Autodesk Inventor part; units mm, degrees
(part 2 of 4)
  line L887 (-15.9707, 10.3342) -> (-15.9954, 10.3717)
  line L888 (-15.9954, 10.3717) -> (-16.0287, 10.4125)
  line L889 (-16.0287, 10.4125) -> (-16.1438, 10.5298)
  line L890 (-16.1438, 10.5298) -> (-16.2774, 10.6739)
  line L891 (-16.2774, 10.6739) -> (-16.4262, 10.8486)
  line L892 (-16.4262, 10.8486) -> (-16.5875, 11.0549)
  line L893 (-16.5875, 11.0549) -> (-16.7591, 11.2943)
  line L894 (-16.7591, 11.2943) -> (-16.8478, 11.4265)
  line L895 (-16.8478, 11.4265) -> (-16.9387, 11.5685)
  line L896 (-16.9387, 11.5685) -> (-17.0299, 11.7175)
  line L897 (-17.0299, 11.7175) -> (-17.1238, 11.8785)
  line L898 (-17.1238, 11.8785) -> (-17.2101, 12.0338)
  arc A26 (-16.763, 12.6491) -> (-17.2101, 12.0338) centre (0, 0) ccw
  line L899 (-16.763, 12.6491) -> (-16.5887, 12.615)
  line L900 (-16.5887, 12.615) -> (-16.4066, 12.5755)
  line L901 (-16.4066, 12.5755) -> (-16.2367, 12.5348)
  line L902 (-16.2367, 12.5348) -> (-16.0735, 12.4922)
  line L903 (-16.0735, 12.4922) -> (-15.9204, 12.4487)
  line L904 (-15.9204, 12.4487) -> (-15.6397, 12.3595)
  line L905 (-15.6397, 12.3595) -> (-15.3936, 12.2698)
  line L906 (-15.3936, 12.2698) -> (-15.1815, 12.1823)
  line L907 (-15.1815, 12.1823) -> (-15.0031, 12.0998)
  line L908 (-15.0031, 12.0998) -> (-14.856, 12.0266)
  line L909 (-14.856, 12.0266) -> (-14.8069, 12.0075)
  line L910 (-14.8069, 12.0075) -> (-14.7636, 11.9956)
  line L911 (-14.7636, 11.9956) -> (-14.7265, 11.9906)
  line L912 (-14.7265, 11.9906) -> (-14.6957, 11.9923)
  line L913 (-14.6957, 11.9923) -> (-14.6716, 12.0004)
  line L914 (-14.6716, 12.0004) -> (-14.6544, 12.0147)
  line L915 (-14.6544, 12.0147) -> (-14.633, 12.0408)
  line L916 (-14.633, 12.0408) -> (-14.4097, 12.307)
  line L917 (-14.4097, 12.307) -> (-14.1816, 12.5693)
  line L918 (-14.1816, 12.5693) -> (-14.1592, 12.5944)
  line L919 (-14.1592, 12.5944) -> (-14.1478, 12.6137)
  line L920 (-14.1478, 12.6137) -> (-14.1436, 12.6387)
  line L921 (-14.1436, 12.6387) -> (-14.1467, 12.6694)
  line L922 (-14.1467, 12.6694) -> (-14.1574, 12.7053)
  line L923 (-14.1574, 12.7053) -> (-14.1759, 12.7462)
  line L924 (-14.1759, 12.7462) -> (-14.2025, 12.7918)
  line L925 (-14.2025, 12.7918) -> (-14.2978, 12.9256)
  line L926 (-14.2978, 12.9256) -> (-14.4072, 13.0888)
  line L927 (-14.4072, 13.0888) -> (-14.5269, 13.2846)
  line L928 (-14.5269, 13.2846) -> (-14.654, 13.5137)
  line L929 (-14.654, 13.5137) -> (-14.786, 13.777)
  line L930 (-14.786, 13.777) -> (-14.8529, 13.9214)
  line L931 (-14.8529, 13.9214) -> (-14.9205, 14.0759)
  line L932 (-14.9205, 14.0759) -> (-14.9872, 14.2373)
  line L933 (-14.9872, 14.2373) -> (-15.0547, 14.411)
  line L934 (-15.0547, 14.411) -> (-15.1157, 14.5779)
  arc A27 (-14.5779, 15.1157) -> (-15.1157, 14.5779) centre (0, 0) ccw
  line L935 (-14.5779, 15.1157) -> (-14.411, 15.0547)
  line L936 (-14.411, 15.0547) -> (-14.2373, 14.9872)
  line L937 (-14.2373, 14.9872) -> (-14.0759, 14.9205)
  line L938 (-14.0759, 14.9205) -> (-13.9214, 14.8528)
  line L939 (-13.9214, 14.8528) -> (-13.777, 14.786)
  line L940 (-13.777, 14.786) -> (-13.5137, 14.6539)
  line L941 (-13.5137, 14.6539) -> (-13.2846, 14.5269)
  line L942 (-13.2846, 14.5269) -> (-13.0888, 14.4072)
  line L943 (-13.0888, 14.4072) -> (-12.9256, 14.2978)
  line L944 (-12.9256, 14.2978) -> (-12.7918, 14.2025)
  line L945 (-12.7918, 14.2025) -> (-12.7462, 14.1759)
  line L946 (-12.7462, 14.1759) -> (-12.7053, 14.1574)
  line L947 (-12.7053, 14.1574) -> (-12.6694, 14.1467)
  line L948 (-12.6694, 14.1467) -> (-12.6387, 14.1436)
  line L949 (-12.6387, 14.1436) -> (-12.6137, 14.1478)
  line L950 (-12.6137, 14.1478) -> (-12.5944, 14.1592)
  line L951 (-12.5944, 14.1592) -> (-12.5693, 14.1816)
  line L952 (-12.5693, 14.1816) -> (-12.307, 14.4097)
  line L953 (-12.307, 14.4097) -> (-12.0408, 14.633)
  line L954 (-12.0408, 14.633) -> (-12.0147, 14.6544)
  line L955 (-12.0147, 14.6544) -> (-12.0004, 14.6716)
  line L956 (-12.0004, 14.6716) -> (-11.9923, 14.6957)
  line L957 (-11.9923, 14.6957) -> (-11.9906, 14.7264)
  line L958 (-11.9906, 14.7264) -> (-11.9956, 14.7636)
  line L959 (-11.9956, 14.7636) -> (-12.0075, 14.8069)
  line L960 (-12.0075, 14.8069) -> (-12.0266, 14.856)
  line L961 (-12.0266, 14.856) -> (-12.0998, 15.0031)
  line L962 (-12.0998, 15.0031) -> (-12.1823, 15.1815)
  line L963 (-12.1823, 15.1815) -> (-12.2698, 15.3936)
  line L964 (-12.2698, 15.3936) -> (-12.3595, 15.6397)
  line L965 (-12.3595, 15.6397) -> (-12.4487, 15.9204)
  line L966 (-12.4487, 15.9204) -> (-12.4922, 16.0735)
  line L967 (-12.4922, 16.0735) -> (-12.5348, 16.2367)
  line L968 (-12.5348, 16.2367) -> (-12.5755, 16.4066)
  line L969 (-12.5755, 16.4066) -> (-12.615, 16.5887)
  line L970 (-12.615, 16.5887) -> (-12.6491, 16.763)
  arc A28 (-12.0338, 17.2101) -> (-12.6491, 16.763) centre (0, 0) ccw
  line L971 (-12.0338, 17.2101) -> (-11.8785, 17.1238)
  line L972 (-11.8785, 17.1238) -> (-11.7175, 17.0299)
  line L973 (-11.7175, 17.0299) -> (-11.5685, 16.9387)
  line L974 (-11.5685, 16.9387) -> (-11.4265, 16.8478)
  line L975 (-11.4265, 16.8478) -> (-11.2943, 16.7591)
  line L976 (-11.2943, 16.7591) -> (-11.0549, 16.5875)
  line L977 (-11.0549, 16.5875) -> (-10.8486, 16.4262)
  line L978 (-10.8486, 16.4262) -> (-10.6739, 16.2774)
  line L979 (-10.6739, 16.2774) -> (-10.5298, 16.1438)
  line L980 (-10.5298, 16.1438) -> (-10.4125, 16.0287)
  line L981 (-10.4125, 16.0287) -> (-10.3717, 15.9954)
  line L982 (-10.3717, 15.9954) -> (-10.3342, 15.9707)
  line L983 (-10.3342, 15.9707) -> (-10.3004, 15.9544)
  line L984 (-10.3004, 15.9544) -> (-10.2706, 15.9466)
  line L985 (-10.2706, 15.9466) -> (-10.2452, 15.9468)
  line L986 (-10.2452, 15.9468) -> (-10.2244, 15.9551)
  line L987 (-10.2244, 15.9551) -> (-10.196, 15.9733)
  line L988 (-10.196, 15.9733) -> (-9.9013, 16.1575)
  line L989 (-9.9013, 16.1575) -> (-9.6034, 16.3364)
  line L990 (-9.6034, 16.3364) -> (-9.5743, 16.3534)
  line L991 (-9.5743, 16.3534) -> (-9.5575, 16.3682)
  line L992 (-9.5575, 16.3682) -> (-9.5457, 16.3908)
  line L993 (-9.5457, 16.3908) -> (-9.5392, 16.4209)
  line L994 (-9.5392, 16.4209) -> (-9.5383, 16.4584)
  line L995 (-9.5383, 16.4584) -> (-9.5433, 16.503)
  line L996 (-9.5433, 16.503) -> (-9.5545, 16.5545)
  line L997 (-9.5545, 16.5545) -> (-9.6038, 16.7112)
  line L998 (-9.6038, 16.7112) -> (-9.6574, 16.9003)
  line L999 (-9.6574, 16.9003) -> (-9.7107, 17.1235)
  line L1000 (-9.7107, 17.1235) -> (-9.7608, 17.3806)
  line L1001 (-9.7608, 17.3806) -> (-9.805, 17.6718)
  line L1002 (-9.805, 17.6718) -> (-9.8239, 17.8299)
  line L1003 (-9.8239, 17.8299) -> (-9.8405, 17.9976)
  line L1004 (-9.8405, 17.9976) -> (-9.8541, 18.1718)
  line L1005 (-9.8541, 18.1718) -> (-9.8647, 18.3579)
  line L1006 (-9.8647, 18.3579) -> (-9.8711, 18.5354)
  arc A29 (-9.1934, 18.8807) -> (-9.8711, 18.5354) centre (0, 0) ccw
  line L1007 (-9.1934, 18.8807) -> (-9.0535, 18.7712)
  line L1008 (-9.0535, 18.7712) -> (-8.9092, 18.6532)
  line L1009 (-8.9092, 18.6532) -> (-8.7763, 18.5399)
  line L1010 (-8.7763, 18.5399) -> (-8.6503, 18.4279)
  line L1011 (-8.6503, 18.4279) -> (-8.5336, 18.3196)
  line L1012 (-8.5336, 18.3196) -> (-8.3239, 18.1127)
  line L1013 (-8.3239, 18.1127) -> (-8.1454, 17.921)
  line L1014 (-8.1454, 17.921) -> (-7.9961, 17.7468)
  line L1015 (-7.9961, 17.7468) -> (-7.8747, 17.5923)
  line L1016 (-7.8747, 17.5923) -> (-7.7769, 17.4603)
  line L1017 (-7.7769, 17.4603) -> (-7.7418, 17.4209)
  line L1018 (-7.7418, 17.4209) -> (-7.7086, 17.3907)
  line L1019 (-7.7086, 17.3907) -> (-7.6778, 17.3693)
  line L1020 (-7.6778, 17.3693) -> (-7.6496, 17.3569)
  line L1021 (-7.6496, 17.3569) -> (-7.6244, 17.3532)
  line L1022 (-7.6244, 17.3532) -> (-7.6026, 17.3581)
  line L1023 (-7.6026, 17.3581) -> (-7.5717, 17.3716)
  line L1024 (-7.5717, 17.3716) -> (-7.2519, 17.5075)
  line L1025 (-7.2519, 17.5075) -> (-6.9296, 17.6376)
  line L1026 (-6.9296, 17.6376) -> (-6.8982, 17.6499)
  line L1027 (-6.8982, 17.6499) -> (-6.8793, 17.6618)
  line L1028 (-6.8793, 17.6618) -> (-6.8641, 17.6822)
  line L1029 (-6.8641, 17.6822) -> (-6.853, 17.711)
  line L1030 (-6.853, 17.711) -> (-6.8462, 17.7479)
  line L1031 (-6.8462, 17.7479) -> (-6.8442, 17.7927)
  line L1032 (-6.8442, 17.7927) -> (-6.8472, 17.8453)
  line L1033 (-6.8472, 17.8453) -> (-6.8714, 18.0078)
  line L1034 (-6.8714, 18.0078) -> (-6.8947, 18.203)
  line L1035 (-6.8947, 18.203) -> (-6.9124, 18.4318)
  line L1036 (-6.9124, 18.4318) -> (-6.9217, 18.6935)
  line L1037 (-6.9217, 18.6935) -> (-6.9198, 18.9881)
  line L1038 (-6.9198, 18.9881) -> (-6.9138, 19.1471)
  line L1039 (-6.9138, 19.1471) -> (-6.9039, 19.3155)
  line L1040 (-6.9039, 19.3155) -> (-6.8901, 19.4896)
  line L1041 (-6.8901, 19.4896) -> (-6.8714, 19.675)
  line L1042 (-6.8714, 19.675) -> (-6.85, 19.8514)
  arc A30 (-6.1266, 20.0864) -> (-6.85, 19.8514) centre (0, 0) ccw
  line L1043 (-6.1266, 20.0864) -> (-6.0056, 19.9563)
  line L1044 (-6.0056, 19.9563) -> (-5.8815, 19.8173)
  line L1045 (-5.8815, 19.8173) -> (-5.7679, 19.6846)
  line L1046 (-5.7679, 19.6846) -> (-5.661, 19.5542)
  line L1047 (-5.661, 19.5542) -> (-5.5627, 19.429)
  line L1048 (-5.5627, 19.429) -> (-5.388, 19.1918)
  line L1049 (-5.388, 19.1918) -> (-5.2416, 18.9746)
  line L1050 (-5.2416, 18.9746) -> (-5.1215, 18.7791)
  line L1051 (-5.1215, 18.7791) -> (-5.0257, 18.6076)
  line L1052 (-5.0257, 18.6076) -> (-4.9497, 18.4619)
  line L1053 (-4.9497, 18.4619) -> (-4.9212, 18.4175)
  line L1054 (-4.9212, 18.4175) -> (-4.8932, 18.3824)
  line L1055 (-4.8932, 18.3824) -> (-4.8661, 18.3566)
  line L1056 (-4.8661, 18.3566) -> (-4.8402, 18.3399)
  line L1057 (-4.8402, 18.3399) -> (-4.8159, 18.3323)
  line L1058 (-4.8159, 18.3323) -> (-4.7936, 18.3337)
  line L1059 (-4.7936, 18.3337) -> (-4.761, 18.3422)
  line L1060 (-4.761, 18.3422) -> (-4.4238, 18.4264)
  line L1061 (-4.4238, 18.4264) -> (-4.0852, 18.5045)
  line L1062 (-4.0852, 18.5045) -> (-4.0522, 18.5117)
  line L1063 (-4.0522, 18.5117) -> (-4.0317, 18.5205)
  line L1064 (-4.0317, 18.5205) -> (-4.0135, 18.5383)
  line L1065 (-4.0135, 18.5383) -> (-3.998, 18.565)
  line L1066 (-3.998, 18.565) -> (-3.9856, 18.6003)
  line L1067 (-3.9856, 18.6003) -> (-3.9765, 18.6443)
  line L1068 (-3.9765, 18.6443) -> (-3.9713, 18.6968)
  line L1069 (-3.9713, 18.6968) -> (-3.9697, 18.8611)
  line L1070 (-3.9697, 18.8611) -> (-3.9623, 19.0574)
  line L1071 (-3.9623, 19.0574) -> (-3.944, 19.2862)
  line L1072 (-3.944, 19.2862) -> (-3.9122, 19.5462)
  line L1073 (-3.9122, 19.5462) -> (-3.8642, 19.8368)
  line L1074 (-3.8642, 19.8368) -> (-3.8334, 19.993)
  line L1075 (-3.8334, 19.993) -> (-3.7973, 20.1577)
  line L1076 (-3.7973, 20.1577) -> (-3.7564, 20.3275)
  line L1077 (-3.7564, 20.3275) -> (-3.7089, 20.5077)
  line L1078 (-3.7089, 20.5077) -> (-3.6602, 20.6786)
  arc A31 (-2.909, 20.7975) -> (-3.6602, 20.6786) centre (0, 0) ccw
  line L1079 (-2.909, 20.7975) -> (-2.8098, 20.6501)
  line L1080 (-2.8098, 20.6501) -> (-2.709, 20.4934)
  line L1081 (-2.709, 20.4934) -> (-2.6176, 20.3445)
  line L1082 (-2.6176, 20.3445) -> (-2.5324, 20.199)
  line L1083 (-2.5324, 20.199) -> (-2.4548, 20.06)
  line L1084 (-2.4548, 20.06) -> (-2.3194, 19.7984)
  line L1085 (-2.3194, 19.7984) -> (-2.2088, 19.561)
  line L1086 (-2.2088, 19.561) -> (-2.1207, 19.3491)
  line L1087 (-2.1207, 19.3491) -> (-2.0529, 19.1647)
  line L1088 (-2.0529, 19.1647) -> (-2.0007, 19.0089)
  line L1089 (-2.0007, 19.0089) -> (-1.9795, 18.9606)
  line L1090 (-1.9795, 18.9606) -> (-1.9573, 18.9216)
  line L1091 (-1.9573, 18.9216) -> (-1.9346, 18.8918)
  line L1092 (-1.9346, 18.8918) -> (-1.9116, 18.8712)
  line L1093 (-1.9116, 18.8712) -> (-1.8888, 18.8599)
  line L1094 (-1.8888, 18.8599) -> (-1.8665, 18.8579)
  line L1095 (-1.8665, 18.8579) -> (-1.833, 18.8612)
  line L1096 (-1.833, 18.8612) -> (-1.4868, 18.8916)
  line L1097 (-1.4868, 18.8916) -> (-1.1401, 18.9157)
  line L1098 (-1.1401, 18.9157) -> (-1.1065, 18.9177)
  line L1099 (-1.1065, 18.9177) -> (-1.0848, 18.9232)
  line L1100 (-1.0848, 18.9232) -> (-1.0641, 18.938)
  line L1101 (-1.0641, 18.938) -> (-1.0446, 18.9618)
  line L1102 (-1.0446, 18.9618) -> (-1.0268, 18.9948)
  line L1103 (-1.0268, 18.9948) -> (-1.011, 19.0368)
  line L1104 (-1.011, 19.0368) -> (-0.9976, 19.0878)
  line L1105 (-0.9976, 19.0878) -> (-0.9703, 19.2499)
  line L1106 (-0.9703, 19.2499) -> (-0.9323, 19.4426)
  line L1107 (-0.9323, 19.4426) -> (-0.8784, 19.6657)
  line L1108 (-0.8784, 19.6657) -> (-0.8063, 19.9175)
  line L1109 (-0.8063, 19.9175) -> (-0.7135, 20.1971)
  line L1110 (-0.7135, 20.1971) -> (-0.6586, 20.3465)
  line L1111 (-0.6586, 20.3465) -> (-0.5972, 20.5035)
  line L1112 (-0.5972, 20.5035) -> (-0.5302, 20.6648)
  line L1113 (-0.5302, 20.6648) -> (-0.4552, 20.8354)
  line L1114 (-0.4552, 20.8354) -> (-0.3803, 20.9966)
  arc A32 (0.3803, 20.9966) -> (-0.3803, 20.9966) centre (0, 0) ccw
  line L1115 (0.3803, 20.9966) -> (0.4552, 20.8354)
  line L1116 (0.4552, 20.8354) -> (0.5302, 20.6648)
  line L1117 (0.5302, 20.6648) -> (0.5972, 20.5035)
  line L1118 (0.5972, 20.5035) -> (0.6586, 20.3465)
  line L1119 (0.6586, 20.3465) -> (0.7135, 20.1971)
  line L1120 (0.7135, 20.1971) -> (0.8063, 19.9175)
  line L1121 (0.8063, 19.9175) -> (0.8784, 19.6657)
  line L1122 (0.8784, 19.6657) -> (0.9323, 19.4426)
  line L1123 (0.9323, 19.4426) -> (0.9703, 19.2499)
  line L1124 (0.9703, 19.2499) -> (0.9976, 19.0878)
  line L1125 (0.9976, 19.0878) -> (1.011, 19.0368)
  line L1126 (1.011, 19.0368) -> (1.0268, 18.9948)
  line L1127 (1.0268, 18.9948) -> (1.0446, 18.9618)
  line L1128 (1.0446, 18.9618) -> (1.0641, 18.938)
  line L1129 (1.0641, 18.938) -> (1.0848, 18.9232)
  line L1130 (1.0848, 18.9232) -> (1.1065, 18.9177)
  line L1131 (1.1065, 18.9177) -> (1.1401, 18.9157)
  line L1132 (1.1401, 18.9157) -> (1.4868, 18.8916)
  line L1133 (1.4868, 18.8916) -> (1.833, 18.8612)
  line L1134 (1.833, 18.8612) -> (1.8665, 18.8579)
  line L1135 (1.8665, 18.8579) -> (1.8888, 18.8599)
  line L1136 (1.8888, 18.8599) -> (1.9116, 18.8712)
  line L1137 (1.9116, 18.8712) -> (1.9346, 18.8918)
  line L1138 (1.9346, 18.8918) -> (1.9573, 18.9216)
  line L1139 (1.9573, 18.9216) -> (1.9795, 18.9606)
  line L1140 (1.9795, 18.9606) -> (2.0007, 19.0089)
  line L1141 (2.0007, 19.0089) -> (2.053, 19.1647)
  line L1142 (2.053, 19.1647) -> (2.1207, 19.3491)
  line L1143 (2.1207, 19.3491) -> (2.2088, 19.561)
  line L1144 (2.2088, 19.561) -> (2.3194, 19.7984)
  line L1145 (2.3194, 19.7984) -> (2.4548, 20.06)
  line L1146 (2.4548, 20.06) -> (2.5324, 20.199)
  line L1147 (2.5324, 20.199) -> (2.6176, 20.3445)
  line L1148 (2.6176, 20.3445) -> (2.709, 20.4934)
  line L1149 (2.709, 20.4934) -> (2.8098, 20.6501)
  line L1150 (2.8098, 20.6501) -> (2.909, 20.7975)
  arc A33 (3.6602, 20.6786) -> (2.909, 20.7975) centre (0, 0) ccw
  line L1151 (3.6602, 20.6786) -> (3.709, 20.5077)
  line L1152 (3.709, 20.5077) -> (3.7564, 20.3275)
  line L1153 (3.7564, 20.3275) -> (3.7973, 20.1577)
  line L1154 (3.7973, 20.1577) -> (3.8334, 19.993)
  line L1155 (3.8334, 19.993) -> (3.8642, 19.8368)
  line L1156 (3.8642, 19.8368) -> (3.9122, 19.5462)
  line L1157 (3.9122, 19.5462) -> (3.944, 19.2862)
  line L1158 (3.944, 19.2862) -> (3.9623, 19.0574)
  line L1159 (3.9623, 19.0574) -> (3.9697, 18.8611)
  line L1160 (3.9697, 18.8611) -> (3.9713, 18.6968)
  line L1161 (3.9713, 18.6968) -> (3.9765, 18.6443)
  line L1162 (3.9765, 18.6443) -> (3.9856, 18.6003)
  line L1163 (3.9856, 18.6003) -> (3.998, 18.565)
  line L1164 (3.998, 18.565) -> (4.0135, 18.5383)
  line L1165 (4.0135, 18.5383) -> (4.0317, 18.5205)
  line L1166 (4.0317, 18.5205) -> (4.0522, 18.5117)
  line L1167 (4.0522, 18.5117) -> (4.0852, 18.5045)
  line L1168 (4.0852, 18.5045) -> (4.4238, 18.4264)
  line L1169 (4.4238, 18.4264) -> (4.761, 18.3422)
  line L1170 (4.761, 18.3422) -> (4.7936, 18.3337)
  line L1171 (4.7936, 18.3337) -> (4.8159, 18.3323)
  line L1172 (4.8159, 18.3323) -> (4.8402, 18.3399)
  line L1173 (4.8402, 18.3399) -> (4.8661, 18.3566)
  line L1174 (4.8661, 18.3566) -> (4.8932, 18.3824)
  line L1175 (4.8932, 18.3824) -> (4.9212, 18.4175)
  line L1176 (4.9212, 18.4175) -> (4.9497, 18.4619)
  line L1177 (4.9497, 18.4619) -> (5.0257, 18.6076)
  line L1178 (5.0257, 18.6076) -> (5.1215, 18.7791)
  line L1179 (5.1215, 18.7791) -> (5.2416, 18.9746)
  line L1180 (5.2416, 18.9746) -> (5.388, 19.1918)
  line L1181 (5.388, 19.1918) -> (5.5627, 19.429)
  line L1182 (5.5627, 19.429) -> (5.661, 19.5542)
  line L1183 (5.661, 19.5542) -> (5.768, 19.6846)
  line L1184 (5.768, 19.6846) -> (5.8815, 19.8173)
  line L1185 (5.8815, 19.8173) -> (6.0056, 19.9563)
  line L1186 (6.0056, 19.9563) -> (6.1266, 20.0864)
  arc A34 (6.85, 19.8514) -> (6.1266, 20.0864) centre (0, 0) ccw
  line L1187 (6.85, 19.8514) -> (6.8714, 19.675)
  line L1188 (6.8714, 19.675) -> (6.8901, 19.4896)
  line L1189 (6.8901, 19.4896) -> (6.9039, 19.3155)
  line L1190 (6.9039, 19.3155) -> (6.9138, 19.1471)
  line L1191 (6.9138, 19.1471) -> (6.9198, 18.9881)
  line L1192 (6.9198, 18.9881) -> (6.9217, 18.6935)
  line L1193 (6.9217, 18.6935) -> (6.9124, 18.4318)
  line L1194 (6.9124, 18.4318) -> (6.8947, 18.203)
  line L1195 (6.8947, 18.203) -> (6.8714, 18.0078)
  line L1196 (6.8714, 18.0078) -> (6.8472, 17.8453)
  line L1197 (6.8472, 17.8453) -> (6.8442, 17.7927)
  line L1198 (6.8442, 17.7927) -> (6.8462, 17.7479)
  line L1199 (6.8462, 17.7479) -> (6.853, 17.711)
  line L1200 (6.853, 17.711) -> (6.8641, 17.6822)
  line L1201 (6.8641, 17.6822) -> (6.8793, 17.6618)
  line L1202 (6.8793, 17.6618) -> (6.8982, 17.6499)
  line L1203 (6.8982, 17.6499) -> (6.9296, 17.6376)
  line L1204 (6.9296, 17.6376) -> (7.2519, 17.5075)
  line L1205 (7.2519, 17.5075) -> (7.5717, 17.3716)
  line L1206 (7.5717, 17.3716) -> (7.6026, 17.3581)
  line L1207 (7.6026, 17.3581) -> (7.6244, 17.3532)
  line L1208 (7.6244, 17.3532) -> (7.6496, 17.3569)
  line L1209 (7.6496, 17.3569) -> (7.6778, 17.3693)
  line L1210 (7.6778, 17.3693) -> (7.7086, 17.3907)
  line L1211 (7.7086, 17.3907) -> (7.7418, 17.4209)
  line L1212 (7.7418, 17.4209) -> (7.7769, 17.4603)
  line L1213 (7.7769, 17.4603) -> (7.8747, 17.5923)
  line L1214 (7.8747, 17.5923) -> (7.9961, 17.7468)
  line L1215 (7.9961, 17.7468) -> (8.1454, 17.921)
  line L1216 (8.1454, 17.921) -> (8.324, 18.1127)
  line L1217 (8.324, 18.1127) -> (8.5336, 18.3196)
  line L1218 (8.5336, 18.3196) -> (8.6503, 18.4279)
  line L1219 (8.6503, 18.4279) -> (8.7763, 18.5399)
  line L1220 (8.7763, 18.5399) -> (8.9092, 18.6532)
  line L1221 (8.9092, 18.6532) -> (9.0535, 18.7712)
  line L1222 (9.0535, 18.7712) -> (9.1934, 18.8807)
  arc A35 (9.8711, 18.5354) -> (9.1934, 18.8807) centre (0, 0) ccw
  line L1223 (9.8711, 18.5354) -> (9.8647, 18.3579)
  line L1224 (9.8647, 18.3579) -> (9.8541, 18.1718)
  line L1225 (9.8541, 18.1718) -> (9.8405, 17.9976)
  line L1226 (9.8405, 17.9976) -> (9.8239, 17.8299)
  line L1227 (9.8239, 17.8299) -> (9.805, 17.6718)
  line L1228 (9.805, 17.6718) -> (9.7608, 17.3806)
  line L1229 (9.7608, 17.3806) -> (9.7107, 17.1235)
  line L1230 (9.7107, 17.1235) -> (9.6574, 16.9003)
  line L1231 (9.6574, 16.9003) -> (9.6038, 16.7112)
  line L1232 (9.6038, 16.7112) -> (9.5545, 16.5545)
  line L1233 (9.5545, 16.5545) -> (9.5433, 16.503)
  line L1234 (9.5433, 16.503) -> (9.5383, 16.4584)
  line L1235 (9.5383, 16.4584) -> (9.5392, 16.4209)
  line L1236 (9.5392, 16.4209) -> (9.5457, 16.3908)
  line L1237 (9.5457, 16.3908) -> (9.5575, 16.3682)
  line L1238 (9.5575, 16.3682) -> (9.5743, 16.3534)
  line L1239 (9.5743, 16.3534) -> (9.6034, 16.3364)
  line L1240 (9.6034, 16.3364) -> (9.9014, 16.1575)
  line L1241 (9.9014, 16.1575) -> (10.196, 15.9733)
  line L1242 (10.196, 15.9733) -> (10.2244, 15.9551)
  line L1243 (10.2244, 15.9551) -> (10.2452, 15.9468)
  line L1244 (10.2452, 15.9468) -> (10.2706, 15.9466)
  line L1245 (10.2706, 15.9466) -> (10.3004, 15.9544)
  line L1246 (10.3004, 15.9544) -> (10.3342, 15.9707)
  line L1247 (10.3342, 15.9707) -> (10.3717, 15.9954)
  line L1248 (10.3717, 15.9954) -> (10.4125, 16.0287)
  line L1249 (10.4125, 16.0287) -> (10.5298, 16.1438)
  line L1250 (10.5298, 16.1438) -> (10.6739, 16.2774)
  line L1251 (10.6739, 16.2774) -> (10.8486, 16.4262)
  line L1252 (10.8486, 16.4262) -> (11.0549, 16.5875)
  line L1253 (11.0549, 16.5875) -> (11.2943, 16.7591)
  line L1254 (11.2943, 16.7591) -> (11.4265, 16.8478)
  line L1255 (11.4265, 16.8478) -> (11.5685, 16.9387)
  line L1256 (11.5685, 16.9387) -> (11.7175, 17.0299)
  line L1257 (11.7175, 17.0299) -> (11.8785, 17.1238)
  line L1258 (11.8785, 17.1238) -> (12.0338, 17.2101)
  arc A36 (12.6491, 16.763) -> (12.0338, 17.2101) centre (0, 0) ccw
  line L1259 (12.6491, 16.763) -> (12.615, 16.5887)
  line L1260 (12.615, 16.5887) -> (12.5755, 16.4066)
  line L1261 (12.5755, 16.4066) -> (12.5348, 16.2367)
  line L1262 (12.5348, 16.2367) -> (12.4922, 16.0735)
  line L1263 (12.4922, 16.0735) -> (12.4487, 15.9204)
  line L1264 (12.4487, 15.9204) -> (12.3595, 15.6397)
  line L1265 (12.3595, 15.6397) -> (12.2698, 15.3936)
  line L1266 (12.2698, 15.3936) -> (12.1823, 15.1815)
  line L1267 (12.1823, 15.1815) -> (12.0998, 15.0031)
  line L1268 (12.0998, 15.0031) -> (12.0266, 14.856)
  line L1269 (12.0266, 14.856) -> (12.0075, 14.8069)
  line L1270 (12.0075, 14.8069) -> (11.9956, 14.7636)
  line L1271 (11.9956, 14.7636) -> (11.9906, 14.7264)
  line L1272 (11.9906, 14.7264) -> (11.9923, 14.6957)
  line L1273 (11.9923, 14.6957) -> (12.0004, 14.6716)
  line L1274 (12.0004, 14.6716) -> (12.0147, 14.6544)
  line L1275 (12.0147, 14.6544) -> (12.0408, 14.633)
  line L1276 (12.0408, 14.633) -> (12.307, 14.4097)
  line L1277 (12.307, 14.4097) -> (12.5693, 14.1816)
  line L1278 (12.5693, 14.1816) -> (12.5944, 14.1592)
  line L1279 (12.5944, 14.1592) -> (12.6137, 14.1478)
  line L1280 (12.6137, 14.1478) -> (12.6388, 14.1436)
  line L1281 (12.6388, 14.1436) -> (12.6694, 14.1467)
  line L1282 (12.6694, 14.1467) -> (12.7053, 14.1574)
  line L1283 (12.7053, 14.1574) -> (12.7462, 14.1759)
  line L1284 (12.7462, 14.1759) -> (12.7918, 14.2025)
  line L1285 (12.7918, 14.2025) -> (12.9256, 14.2978)
  line L1286 (12.9256, 14.2978) -> (13.0888, 14.4072)
  line L1287 (13.0888, 14.4072) -> (13.2846, 14.5269)
  line L1288 (13.2846, 14.5269) -> (13.5137, 14.6539)
  line L1289 (13.5137, 14.6539) -> (13.777, 14.786)
  line L1290 (13.777, 14.786) -> (13.9214, 14.8528)
  line L1291 (13.9214, 14.8528) -> (14.0759, 14.9205)
  line L1292 (14.0759, 14.9205) -> (14.2373, 14.9872)
  line L1293 (14.2373, 14.9872) -> (14.411, 15.0547)
  line L1294 (14.411, 15.0547) -> (14.5779, 15.1157)
  arc A37 (15.1157, 14.5779) -> (14.5779, 15.1157) centre (0, 0) ccw
  line L1295 (15.1157, 14.5779) -> (15.0547, 14.411)
  line L1296 (15.0547, 14.411) -> (14.9872, 14.2373)
  line L1297 (14.9872, 14.2373) -> (14.9205, 14.0759)
  line L1298 (14.9205, 14.0759) -> (14.8529, 13.9214)
  line L1299 (14.8529, 13.9214) -> (14.786, 13.777)
  line L1300 (14.786, 13.777) -> (14.654, 13.5137)
  line L1301 (14.654, 13.5137) -> (14.5269, 13.2846)
  line L1302 (14.5269, 13.2846) -> (14.4072, 13.0888)
  line L1303 (14.4072, 13.0888) -> (14.2978, 12.9256)
  line L1304 (14.2978, 12.9256) -> (14.2025, 12.7918)
  line L1305 (14.2025, 12.7918) -> (14.1759, 12.7462)
  line L1306 (14.1759, 12.7462) -> (14.1574, 12.7053)
  line L1307 (14.1574, 12.7053) -> (14.1467, 12.6694)
  line L1308 (14.1467, 12.6694) -> (14.1436, 12.6387)
  line L1309 (14.1436, 12.6387) -> (14.1478, 12.6137)
  line L1310 (14.1478, 12.6137) -> (14.1592, 12.5944)
  line L1311 (14.1592, 12.5944) -> (14.1816, 12.5693)
  line L1312 (14.1816, 12.5693) -> (14.4097, 12.307)
  line L1313 (14.4097, 12.307) -> (14.633, 12.0408)
  line L1314 (14.633, 12.0408) -> (14.6544, 12.0147)
  line L1315 (14.6544, 12.0147) -> (14.6716, 12.0004)
  line L1316 (14.6716, 12.0004) -> (14.6957, 11.9923)
  line L1317 (14.6957, 11.9923) -> (14.7265, 11.9906)
  line L1318 (14.7265, 11.9906) -> (14.7636, 11.9956)
  line L1319 (14.7636, 11.9956) -> (14.8069, 12.0075)
  line L1320 (14.8069, 12.0075) -> (14.856, 12.0266)
  line L1321 (14.856, 12.0266) -> (15.0031, 12.0998)
  line L1322 (15.0031, 12.0998) -> (15.1815, 12.1823)
  line L1323 (15.1815, 12.1823) -> (15.3936, 12.2698)
  line L1324 (15.3936, 12.2698) -> (15.6397, 12.3595)
  line L1325 (15.6397, 12.3595) -> (15.9204, 12.4487)
  line L1326 (15.9204, 12.4487) -> (16.0735, 12.4922)
  line L1327 (16.0735, 12.4922) -> (16.2367, 12.5348)
  line L1328 (16.2367, 12.5348) -> (16.4066, 12.5755)
  line L1329 (16.4066, 12.5755) -> (16.5887, 12.615)
  line L1330 (16.5887, 12.615) -> (16.7631, 12.6491)
  arc A38 (17.2101, 12.0338) -> (16.7631, 12.6491) centre (0, 0) ccw
  line L1331 (17.2101, 12.0338) -> (17.1238, 11.8785)
  line L1332 (17.1238, 11.8785) -> (17.0299, 11.7175)
  line L1333 (17.0299, 11.7175) -> (16.9387, 11.5685)
  line L1334 (16.9387, 11.5685) -> (16.8478, 11.4265)
  line L1335 (16.8478, 11.4265) -> (16.7591, 11.2943)
  line L1336 (16.7591, 11.2943) -> (16.5875, 11.0549)
  line L1337 (16.5875, 11.0549) -> (16.4262, 10.8486)
  line L1338 (16.4262, 10.8486) -> (16.2774, 10.6739)
  line L1339 (16.2774, 10.6739) -> (16.1438, 10.5298)
  line L1340 (16.1438, 10.5298) -> (16.0287, 10.4125)
  line L1341 (16.0287, 10.4125) -> (15.9954, 10.3717)
  line L1342 (15.9954, 10.3717) -> (15.9707, 10.3342)
  line L1343 (15.9707, 10.3342) -> (15.9544, 10.3004)
  line L1344 (15.9544, 10.3004) -> (15.9466, 10.2706)
  line L1345 (15.9466, 10.2706) -> (15.9468, 10.2452)
  line L1346 (15.9468, 10.2452) -> (15.9551, 10.2244)
  line L1347 (15.9551, 10.2244) -> (15.9733, 10.196)
  line L1348 (15.9733, 10.196) -> (16.1575, 9.9013)
  line L1349 (16.1575, 9.9013) -> (16.3364, 9.6034)
  line L1350 (16.3364, 9.6034) -> (16.3535, 9.5743)
  line L1351 (16.3535, 9.5743) -> (16.3682, 9.5575)
  line L1352 (16.3682, 9.5575) -> (16.3908, 9.5457)
  line L1353 (16.3908, 9.5457) -> (16.4209, 9.5392)
  line L1354 (16.4209, 9.5392) -> (16.4584, 9.5383)
  line L1355 (16.4584, 9.5383) -> (16.503, 9.5433)
  line L1356 (16.503, 9.5433) -> (16.5545, 9.5545)
  line L1357 (16.5545, 9.5545) -> (16.7112, 9.6038)
  line L1358 (16.7112, 9.6038) -> (16.9003, 9.6574)
  line L1359 (16.9003, 9.6574) -> (17.1235, 9.7107)
  line L1360 (17.1235, 9.7107) -> (17.3806, 9.7608)
  line L1361 (17.3806, 9.7608) -> (17.6718, 9.805)
  line L1362 (17.6718, 9.805) -> (17.8299, 9.8239)
  line L1363 (17.8299, 9.8239) -> (17.9976, 9.8405)
  line L1364 (17.9976, 9.8405) -> (18.1718, 9.8541)
  line L1365 (18.1718, 9.8541) -> (18.3579, 9.8646)
  line L1366 (18.3579, 9.8646) -> (18.5354, 9.8711)
  arc A39 (18.8807, 9.1934) -> (18.5354, 9.8711) centre (0, 0) ccw
  line L1367 (18.8807, 9.1934) -> (18.7712, 9.0535)
  line L1368 (18.7712, 9.0535) -> (18.6532, 8.9092)
  line L1369 (18.6532, 8.9092) -> (18.5399, 8.7763)
  line L1370 (18.5399, 8.7763) -> (18.4279, 8.6503)
  line L1371 (18.4279, 8.6503) -> (18.3196, 8.5336)
  line L1372 (18.3196, 8.5336) -> (18.1127, 8.3239)
  line L1373 (18.1127, 8.3239) -> (17.9211, 8.1454)
  line L1374 (17.9211, 8.1454) -> (17.7468, 7.9961)
  line L1375 (17.7468, 7.9961) -> (17.5923, 7.8747)
  line L1376 (17.5923, 7.8747) -> (17.4603, 7.7769)
  line L1377 (17.4603, 7.7769) -> (17.4209, 7.7418)
  line L1378 (17.4209, 7.7418) -> (17.3907, 7.7086)
  line L1379 (17.3907, 7.7086) -> (17.3694, 7.6778)
  line L1380 (17.3694, 7.6778) -> (17.3569, 7.6496)
  line L1381 (17.3569, 7.6496) -> (17.3532, 7.6244)
  line L1382 (17.3532, 7.6244) -> (17.3581, 7.6026)
  line L1383 (17.3581, 7.6026) -> (17.3717, 7.5717)
  line L1384 (17.3717, 7.5717) -> (17.5075, 7.2518)
  line L1385 (17.5075, 7.2518) -> (17.6376, 6.9296)
  line L1386 (17.6376, 6.9296) -> (17.6499, 6.8982)
  line L1387 (17.6499, 6.8982) -> (17.6618, 6.8793)
  line L1388 (17.6618, 6.8793) -> (17.6823, 6.8641)
  line L1389 (17.6823, 6.8641) -> (17.711, 6.853)
  line L1390 (17.711, 6.853) -> (17.7479, 6.8462)
  line L1391 (17.7479, 6.8462) -> (17.7927, 6.8442)
  line L1392 (17.7927, 6.8442) -> (17.8454, 6.8472)
  line L1393 (17.8454, 6.8472) -> (18.0079, 6.8714)
  line L1394 (18.0079, 6.8714) -> (18.203, 6.8947)
  line L1395 (18.203, 6.8947) -> (18.4318, 6.9124)
  line L1396 (18.4318, 6.9124) -> (18.6935, 6.9217)
  line L1397 (18.6935, 6.9217) -> (18.9881, 6.9198)
  line L1398 (18.9881, 6.9198) -> (19.1472, 6.9138)
  line L1399 (19.1472, 6.9138) -> (19.3155, 6.9039)
  line L1400 (19.3155, 6.9039) -> (19.4896, 6.8901)
  line L1401 (19.4896, 6.8901) -> (19.675, 6.8714)
  line L1402 (19.675, 6.8714) -> (19.8514, 6.85)
  arc A40 (20.0864, 6.1266) -> (19.8514, 6.85) centre (0, 0) ccw
  line L1403 (20.0864, 6.1266) -> (19.9563, 6.0056)
  line L1404 (19.9563, 6.0056) -> (19.8173, 5.8815)
  line L1405 (19.8173, 5.8815) -> (19.6846, 5.7679)
  line L1406 (19.6846, 5.7679) -> (19.5542, 5.661)
  line L1407 (19.5542, 5.661) -> (19.429, 5.5627)
  line L1408 (19.429, 5.5627) -> (19.1918, 5.388)
  line L1409 (19.1918, 5.388) -> (18.9746, 5.2416)
  line L1410 (18.9746, 5.2416) -> (18.7791, 5.1215)
  line L1411 (18.7791, 5.1215) -> (18.6076, 5.0257)
  line L1412 (18.6076, 5.0257) -> (18.4619, 4.9497)
  line L1413 (18.4619, 4.9497) -> (18.4175, 4.9212)
  line L1414 (18.4175, 4.9212) -> (18.3824, 4.8932)
  line L1415 (18.3824, 4.8932) -> (18.3566, 4.8661)
  line L1416 (18.3566, 4.8661) -> (18.3399, 4.8402)
  line L1417 (18.3399, 4.8402) -> (18.3323, 4.8159)
  line L1418 (18.3323, 4.8159) -> (18.3337, 4.7936)
  line L1419 (18.3337, 4.7936) -> (18.3423, 4.761)
  line L1420 (18.3423, 4.761) -> (18.4264, 4.4238)
  line L1421 (18.4264, 4.4238) -> (18.5045, 4.0851)
  line L1422 (18.5045, 4.0851) -> (18.5117, 4.0522)
  line L1423 (18.5117, 4.0522) -> (18.5205, 4.0317)
  line L1424 (18.5205, 4.0317) -> (18.5383, 4.0135)
  line L1425 (18.5383, 4.0135) -> (18.565, 3.998)
  line L1426 (18.565, 3.998) -> (18.6003, 3.9856)
  line L1427 (18.6003, 3.9856) -> (18.6443, 3.9765)
  line L1428 (18.6443, 3.9765) -> (18.6968, 3.9713)
  line L1429 (18.6968, 3.9713) -> (18.8611, 3.9697)
  line L1430 (18.8611, 3.9697) -> (19.0574, 3.9623)
  line L1431 (19.0574, 3.9623) -> (19.2862, 3.944)
  line L1432 (19.2862, 3.944) -> (19.5462, 3.9122)
  line L1433 (19.5462, 3.9122) -> (19.8368, 3.8642)
  line L1434 (19.8368, 3.8642) -> (19.993, 3.8334)
  line L1435 (19.993, 3.8334) -> (20.1577, 3.7973)
  line L1436 (20.1577, 3.7973) -> (20.3275, 3.7564)
  line L1437 (20.3275, 3.7564) -> (20.5077, 3.7089)
  line L1438 (20.5077, 3.7089) -> (20.6786, 3.6602)
  arc A41 (20.7975, 2.909) -> (20.6786, 3.6602) centre (0, 0) ccw
  line L1439 (20.7975, 2.909) -> (20.6501, 2.8098)
  line L1440 (20.6501, 2.8098) -> (20.4934, 2.709)
  line L1441 (20.4934, 2.709) -> (20.3445, 2.6176)
  line L1442 (20.3445, 2.6176) -> (20.199, 2.5324)
  line L1443 (20.199, 2.5324) -> (20.06, 2.4548)
  line L1444 (20.06, 2.4548) -> (19.7984, 2.3194)
  line L1445 (19.7984, 2.3194) -> (19.561, 2.2088)
  line L1446 (19.561, 2.2088) -> (19.3491, 2.1207)
  line L1447 (19.3491, 2.1207) -> (19.1647, 2.0529)
  line L1448 (19.1647, 2.0529) -> (19.0089, 2.0007)
  line L1449 (19.0089, 2.0007) -> (18.9606, 1.9795)
  line L1450 (18.9606, 1.9795) -> (18.9216, 1.9573)
  line L1451 (18.9216, 1.9573) -> (18.8918, 1.9346)
  line L1452 (18.8918, 1.9346) -> (18.8713, 1.9116)
  line L1453 (18.8713, 1.9116) -> (18.86, 1.8888)
  line L1454 (18.86, 1.8888) -> (18.8579, 1.8665)
  line L1455 (18.8579, 1.8665) -> (18.8612, 1.833)
  line L1456 (18.8612, 1.833) -> (18.8916, 1.4868)
  line L1457 (18.8916, 1.4868) -> (18.9157, 1.1401)
  line L1458 (18.9157, 1.1401) -> (18.9177, 1.1065)
  line L1459 (18.9177, 1.1065) -> (18.9232, 1.0848)
  line L1460 (18.9232, 1.0848) -> (18.938, 1.0641)
  line L1461 (18.938, 1.0641) -> (18.9618, 1.0446)
  line L1462 (18.9618, 1.0446) -> (18.9948, 1.0268)
  line L1463 (18.9948, 1.0268) -> (19.0368, 1.011)
  line L1464 (19.0368, 1.011) -> (19.0878, 0.9976)
  line L1465 (19.0878, 0.9976) -> (19.2499, 0.9703)
  line L1466 (19.2499, 0.9703) -> (19.4426, 0.9323)
  line L1467 (19.4426, 0.9323) -> (19.6657, 0.8784)
  line L1468 (19.6657, 0.8784) -> (19.9175, 0.8063)
  line L1469 (19.9175, 0.8063) -> (20.1971, 0.7134)
  line L1470 (20.1971, 0.7134) -> (20.3465, 0.6586)
  line L1471 (20.3465, 0.6586) -> (20.5035, 0.5972)
  line L1472 (20.5035, 0.5972) -> (20.6649, 0.5302)
  line L1473 (20.6649, 0.5302) -> (20.8354, 0.4552)
  line L1474 (20.8354, 0.4552) -> (20.9966, 0.3803)
  arc A42 (20.9966, -0.3803) -> (20.9966, 0.3803) centre (0, 0) ccw
  line L1475 (20.9966, -0.3803) -> (20.8354, -0.4552)
  line L1476 (20.8354, -0.4552) -> (20.6649, -0.5302)
  line L1477 (20.6649, -0.5302) -> (20.5035, -0.5972)
  line L1478 (20.5035, -0.5972) -> (20.3465, -0.6586)
  line L1479 (20.3465, -0.6586) -> (20.1971, -0.7135)
  line L1480 (20.1971, -0.7135) -> (19.9175, -0.8063)
  line L1481 (19.9175, -0.8063) -> (19.6657, -0.8784)
  line L1482 (19.6657, -0.8784) -> (19.4426, -0.9323)
  line L1483 (19.4426, -0.9323) -> (19.2499, -0.9703)
  line L1484 (19.2499, -0.9703) -> (19.0878, -0.9976)
  line L1485 (19.0878, -0.9976) -> (19.0368, -1.011)
  line L1486 (19.0368, -1.011) -> (18.9948, -1.0268)
  line L1487 (18.9948, -1.0268) -> (18.9618, -1.0446)
  line L1488 (18.9618, -1.0446) -> (18.938, -1.0641)
  line L1489 (18.938, -1.0641) -> (18.9232, -1.0848)
  line L1490 (18.9232, -1.0848) -> (18.9177, -1.1065)
  line L1491 (18.9177, -1.1065) -> (18.9157, -1.1401)
  line L1492 (18.9157, -1.1401) -> (18.8916, -1.4868)
  line L1493 (18.8916, -1.4868) -> (18.8612, -1.833)
  line L1494 (18.8612, -1.833) -> (18.8579, -1.8665)
  line L1495 (18.8579, -1.8665) -> (18.86, -1.8888)
  line L1496 (18.86, -1.8888) -> (18.8713, -1.9116)
  line L1497 (18.8713, -1.9116) -> (18.8918, -1.9346)
  line L1498 (18.8918, -1.9346) -> (18.9216, -1.9573)
  line L1499 (18.9216, -1.9573) -> (18.9606, -1.9795)
  line L1500 (18.9606, -1.9795) -> (19.0089, -2.0007)
  line L1501 (19.0089, -2.0007) -> (19.1647, -2.053)
  line L1502 (19.1647, -2.053) -> (19.3491, -2.1207)
  line L1503 (19.3491, -2.1207) -> (19.561, -2.2088)
  line L1504 (19.561, -2.2088) -> (19.7984, -2.3194)
  line L1505 (19.7984, -2.3194) -> (20.06, -2.4548)
  line L1506 (20.06, -2.4548) -> (20.199, -2.5324)
  line L1507 (20.199, -2.5324) -> (20.3445, -2.6176)
  line L1508 (20.3445, -2.6176) -> (20.4934, -2.709)
  line L1509 (20.4934, -2.709) -> (20.6501, -2.8098)
  line L1510 (20.6501, -2.8098) -> (20.7975, -2.909)
  arc A43 (20.6786, -3.6602) -> (20.7975, -2.909) centre (0, 0) ccw
  line L1511 (20.6786, -3.6602) -> (20.5077, -3.709)
  line L1512 (20.5077, -3.709) -> (20.3275, -3.7564)
  line L1513 (20.3275, -3.7564) -> (20.1577, -3.7973)
  line L1514 (20.1577, -3.7973) -> (19.993, -3.8334)
  line L1515 (19.993, -3.8334) -> (19.8368, -3.8642)
  line L1516 (19.8368, -3.8642) -> (19.5462, -3.9122)
  line L1517 (19.5462, -3.9122) -> (19.2862, -3.944)
  line L1518 (19.2862, -3.944) -> (19.0574, -3.9623)
  line L1519 (19.0574, -3.9623) -> (18.8611, -3.9697)
  line L1520 (18.8611, -3.9697) -> (18.6968, -3.9713)
  line L1521 (18.6968, -3.9713) -> (18.6443, -3.9765)
  line L1522 (18.6443, -3.9765) -> (18.6003, -3.9856)
  line L1523 (18.6003, -3.9856) -> (18.565, -3.998)
  line L1524 (18.565, -3.998) -> (18.5383, -4.0135)
  line L1525 (18.5383, -4.0135) -> (18.5205, -4.0317)
  line L1526 (18.5205, -4.0317) -> (18.5117, -4.0522)
  line L1527 (18.5117, -4.0522) -> (18.5045, -4.0852)
  line L1528 (18.5045, -4.0852) -> (18.4264, -4.4238)
  line L1529 (18.4264, -4.4238) -> (18.3423, -4.761)
  line L1530 (18.3423, -4.761) -> (18.3337, -4.7936)
  line L1531 (18.3337, -4.7936) -> (18.3323, -4.8159)
  line L1532 (18.3323, -4.8159) -> (18.3399, -4.8402)
  line L1533 (18.3399, -4.8402) -> (18.3566, -4.8661)
  line L1534 (18.3566, -4.8661) -> (18.3824, -4.8932)
  line L1535 (18.3824, -4.8932) -> (18.4175, -4.9212)
  line L1536 (18.4175, -4.9212) -> (18.4619, -4.9497)
  line L1537 (18.4619, -4.9497) -> (18.6076, -5.0257)
  line L1538 (18.6076, -5.0257) -> (18.7791, -5.1215)
  line L1539 (18.7791, -5.1215) -> (18.9746, -5.2416)
  line L1540 (18.9746, -5.2416) -> (19.1918, -5.388)
  line L1541 (19.1918, -5.388) -> (19.429, -5.5627)
  line L1542 (19.429, -5.5627) -> (19.5542, -5.661)
  line L1543 (19.5542, -5.661) -> (19.6846, -5.768)
  line L1544 (19.6846, -5.768) -> (19.8173, -5.8815)
  line L1545 (19.8173, -5.8815) -> (19.9563, -6.0056)
  line L1546 (19.9563, -6.0056) -> (20.0864, -6.1266)
  arc A44 (19.8514, -6.85) -> (20.0864, -6.1266) centre (0, 0) ccw
  line L1547 (19.8514, -6.85) -> (19.675, -6.8714)
  line L1548 (19.675, -6.8714) -> (19.4896, -6.8901)
  line L1549 (19.4896, -6.8901) -> (19.3155, -6.9039)
  line L1550 (19.3155, -6.9039) -> (19.1472, -6.9138)
  line L1551 (19.1472, -6.9138) -> (18.9881, -6.9198)
  line L1552 (18.9881, -6.9198) -> (18.6935, -6.9217)
  line L1553 (18.6935, -6.9217) -> (18.4318, -6.9124)
  line L1554 (18.4318, -6.9124) -> (18.203, -6.8948)
  line L1555 (18.203, -6.8948) -> (18.0079, -6.8714)
  line L1556 (18.0079, -6.8714) -> (17.8454, -6.8472)
  line L1557 (17.8454, -6.8472) -> (17.7927, -6.8442)
  line L1558 (17.7927, -6.8442) -> (17.7479, -6.8462)
  line L1559 (17.7479, -6.8462) -> (17.711, -6.853)
  line L1560 (17.711, -6.853) -> (17.6823, -6.8641)
  line L1561 (17.6823, -6.8641) -> (17.6618, -6.8793)
  line L1562 (17.6618, -6.8793) -> (17.6499, -6.8982)
  line L1563 (17.6499, -6.8982) -> (17.6376, -6.9296)
  line L1564 (17.6376, -6.9296) -> (17.5075, -7.2519)
  line L1565 (17.5075, -7.2519) -> (17.3717, -7.5717)
  line L1566 (17.3717, -7.5717) -> (17.3581, -7.6026)
  line L1567 (17.3581, -7.6026) -> (17.3532, -7.6244)
  line L1568 (17.3532, -7.6244) -> (17.3569, -7.6496)
  line L1569 (17.3569, -7.6496) -> (17.3694, -7.6778)
  line L1570 (17.3694, -7.6778) -> (17.3907, -7.7086)
  line L1571 (17.3907, -7.7086) -> (17.4209, -7.7418)
  line L1572 (17.4209, -7.7418) -> (17.4603, -7.7769)
  line L1573 (17.4603, -7.7769) -> (17.5923, -7.8747)
  line L1574 (17.5923, -7.8747) -> (17.7468, -7.9961)
  line L1575 (17.7468, -7.9961) -> (17.9211, -8.1454)
  line L1576 (17.9211, -8.1454) -> (18.1127, -8.324)
  line L1577 (18.1127, -8.324) -> (18.3196, -8.5336)
  line L1578 (18.3196, -8.5336) -> (18.4279, -8.6503)
  line L1579 (18.4279, -8.6503) -> (18.5399, -8.7763)
  line L1580 (18.5399, -8.7763) -> (18.6532, -8.9092)
  line L1581 (18.6532, -8.9092) -> (18.7712, -9.0535)
  line L1582 (18.7712, -9.0535) -> (18.8807, -9.1934)
  arc A45 (18.5354, -9.8711) -> (18.8807, -9.1934) centre (0, 0) ccw
  line L1583 (18.5354, -9.8711) -> (18.3579, -9.8647)
  line L1584 (18.3579, -9.8647) -> (18.1718, -9.8541)
  line L1585 (18.1718, -9.8541) -> (17.9976, -9.8405)
  line L1586 (17.9976, -9.8405) -> (17.8299, -9.8239)
  line L1587 (17.8299, -9.8239) -> (17.6718, -9.805)
  line L1588 (17.6718, -9.805) -> (17.3806, -9.7608)
  line L1589 (17.3806, -9.7608) -> (17.1235, -9.7107)
  line L1590 (17.1235, -9.7107) -> (16.9003, -9.6574)
  line L1591 (16.9003, -9.6574) -> (16.7112, -9.6038)
  line L1592 (16.7112, -9.6038) -> (16.5545, -9.5545)
  line L1593 (16.5545, -9.5545) -> (16.503, -9.5433)
  line L1594 (16.503, -9.5433) -> (16.4584, -9.5383)
  line L1595 (16.4584, -9.5383) -> (16.4209, -9.5392)
  line L1596 (16.4209, -9.5392) -> (16.3908, -9.5457)
  line L1597 (16.3908, -9.5457) -> (16.3682, -9.5575)
  line L1598 (16.3682, -9.5575) -> (16.3535, -9.5743)
  line L1599 (16.3535, -9.5743) -> (16.3364, -9.6034)
  line L1600 (16.3364, -9.6034) -> (16.1575, -9.9014)
  line L1601 (16.1575, -9.9014) -> (15.9733, -10.196)
  line L1602 (15.9733, -10.196) -> (15.9551, -10.2244)
  line L1603 (15.9551, -10.2244) -> (15.9468, -10.2452)
  line L1604 (15.9468, -10.2452) -> (15.9466, -10.2706)
  line L1605 (15.9466, -10.2706) -> (15.9544, -10.3004)
  line L1606 (15.9544, -10.3004) -> (15.9707, -10.3342)
  line L1607 (15.9707, -10.3342) -> (15.9954, -10.3717)
  line L1608 (15.9954, -10.3717) -> (16.0287, -10.4125)
  line L1609 (16.0287, -10.4125) -> (16.1438, -10.5298)
  line L1610 (16.1438, -10.5298) -> (16.2774, -10.6739)
  line L1611 (16.2774, -10.6739) -> (16.4262, -10.8486)
  line L1612 (16.4262, -10.8486) -> (16.5875, -11.0549)
  line L1613 (16.5875, -11.0549) -> (16.7591, -11.2943)
  line L1614 (16.7591, -11.2943) -> (16.8478, -11.4266)
  line L1615 (16.8478, -11.4266) -> (16.9387, -11.5685)
  line L1616 (16.9387, -11.5685) -> (17.0299, -11.7175)
  line L1617 (17.0299, -11.7175) -> (17.1238, -11.8785)
  line L1618 (17.1238, -11.8785) -> (17.2101, -12.0338)
  arc A46 (16.7631, -12.6491) -> (17.2101, -12.0338) centre (0, 0) ccw
  line L1619 (16.7631, -12.6491) -> (16.5887, -12.615)
  line L1620 (16.5887, -12.615) -> (16.4066, -12.5755)
  line L1621 (16.4066, -12.5755) -> (16.2367, -12.5348)
  line L1622 (16.2367, -12.5348) -> (16.0735, -12.4922)
  line L1623 (16.0735, -12.4922) -> (15.9204, -12.4487)
  line L1624 (15.9204, -12.4487) -> (15.6397, -12.3595)
  line L1625 (15.6397, -12.3595) -> (15.3936, -12.2699)
  line L1626 (15.3936, -12.2699) -> (15.1815, -12.1823)
  line L1627 (15.1815, -12.1823) -> (15.0031, -12.0998)
  line L1628 (15.0031, -12.0998) -> (14.856, -12.0266)
  line L1629 (14.856, -12.0266) -> (14.8069, -12.0075)
  line L1630 (14.8069, -12.0075) -> (14.7636, -11.9956)
  line L1631 (14.7636, -11.9956) -> (14.7265, -11.9906)
  line L1632 (14.7265, -11.9906) -> (14.6957, -11.9923)
  line L1633 (14.6957, -11.9923) -> (14.6716, -12.0004)
  line L1634 (14.6716, -12.0004) -> (14.6544, -12.0147)
  line L1635 (14.6544, -12.0147) -> (14.633, -12.0408)
  line L1636 (14.633, -12.0408) -> (14.4097, -12.307)
  line L1637 (14.4097, -12.307) -> (14.1816, -12.5693)
  line L1638 (14.1816, -12.5693) -> (14.1592, -12.5944)
  line L1639 (14.1592, -12.5944) -> (14.1478, -12.6137)
  line L1640 (14.1478, -12.6137) -> (14.1436, -12.6388)
  line L1641 (14.1436, -12.6388) -> (14.1467, -12.6694)
  line L1642 (14.1467, -12.6694) -> (14.1574, -12.7053)
  line L1643 (14.1574, -12.7053) -> (14.1759, -12.7462)
  line L1644 (14.1759, -12.7462) -> (14.2025, -12.7918)
  line L1645 (14.2025, -12.7918) -> (14.2978, -12.9256)
  line L1646 (14.2978, -12.9256) -> (14.4072, -13.0888)
  line L1647 (14.4072, -13.0888) -> (14.5269, -13.2846)
  line L1648 (14.5269, -13.2846) -> (14.654, -13.5137)
  line L1649 (14.654, -13.5137) -> (14.786, -13.777)
  line L1650 (14.786, -13.777) -> (14.8529, -13.9214)
  line L1651 (14.8529, -13.9214) -> (14.9205, -14.0759)
  line L1652 (14.9205, -14.0759) -> (14.9872, -14.2373)
  line L1653 (14.9872, -14.2373) -> (15.0547, -14.411)
  line L1654 (15.0547, -14.411) -> (15.1157, -14.5779)
  arc A47 (14.5779, -15.1157) -> (15.1157, -14.5779) centre (0, 0) ccw
  line L1655 (14.5779, -15.1157) -> (14.411, -15.0547)
  line L1656 (14.411, -15.0547) -> (14.2373, -14.9872)
  line L1657 (14.2373, -14.9872) -> (14.0759, -14.9205)
  line L1658 (14.0759, -14.9205) -> (13.9214, -14.8529)
  line L1659 (13.9214, -14.8529) -> (13.777, -14.786)
  line L1660 (13.777, -14.786) -> (13.5137, -14.654)
  line L1661 (13.5137, -14.654) -> (13.2846, -14.5269)
  line L1662 (13.2846, -14.5269) -> (13.0888, -14.4072)
  line L1663 (13.0888, -14.4072) -> (12.9256, -14.2978)
  line L1664 (12.9256, -14.2978) -> (12.7918, -14.2025)
  line L1665 (12.7918, -14.2025) -> (12.7462, -14.176)
  line L1666 (12.7462, -14.176) -> (12.7053, -14.1574)
  line L1667 (12.7053, -14.1574) -> (12.6694, -14.1467)
  line L1668 (12.6694, -14.1467) -> (12.6388, -14.1436)
  line L1669 (12.6388, -14.1436) -> (12.6137, -14.1478)
  line L1670 (12.6137, -14.1478) -> (12.5944, -14.1592)
  line L1671 (12.5944, -14.1592) -> (12.5693, -14.1816)
  line L1672 (12.5693, -14.1816) -> (12.307, -14.4097)
  line L1673 (12.307, -14.4097) -> (12.0408, -14.633)
  line L1674 (12.0408, -14.633) -> (12.0147, -14.6544)
  line L1675 (12.0147, -14.6544) -> (12.0004, -14.6716)
  line L1676 (12.0004, -14.6716) -> (11.9923, -14.6957)
  line L1677 (11.9923, -14.6957) -> (11.9906, -14.7265)
  line L1678 (11.9906, -14.7265) -> (11.9956, -14.7636)
  line L1679 (11.9956, -14.7636) -> (12.0075, -14.8069)
  line L1680 (12.0075, -14.8069) -> (12.0266, -14.856)
  line L1681 (12.0266, -14.856) -> (12.0998, -15.0031)
  line L1682 (12.0998, -15.0031) -> (12.1823, -15.1815)
  line L1683 (12.1823, -15.1815) -> (12.2698, -15.3936)
  line L1684 (12.2698, -15.3936) -> (12.3595, -15.6397)
  line L1685 (12.3595, -15.6397) -> (12.4487, -15.9204)
  line L1686 (12.4487, -15.9204) -> (12.4922, -16.0736)
  line L1687 (12.4922, -16.0736) -> (12.5348, -16.2367)
  line L1688 (12.5348, -16.2367) -> (12.5755, -16.4066)
  line L1689 (12.5755, -16.4066) -> (12.615, -16.5887)
  line L1690 (12.615, -16.5887) -> (12.6491, -16.7631)
  arc A48 (12.0338, -17.2101) -> (12.6491, -16.7631) centre (0, 0) ccw
  line L1691 (12.0338, -17.2101) -> (11.8785, -17.1238)
  line L1692 (11.8785, -17.1238) -> (11.7175, -17.0299)
  line L1693 (11.7175, -17.0299) -> (11.5685, -16.9387)
  line L1694 (11.5685, -16.9387) -> (11.4265, -16.8478)
  line L1695 (11.4265, -16.8478) -> (11.2943, -16.7591)
  line L1696 (11.2943, -16.7591) -> (11.0549, -16.5875)
  line L1697 (11.0549, -16.5875) -> (10.8486, -16.4262)
  line L1698 (10.8486, -16.4262) -> (10.6739, -16.2774)
  line L1699 (10.6739, -16.2774) -> (10.5298, -16.1438)
  line L1700 (10.5298, -16.1438) -> (10.4125, -16.0287)
  line L1701 (10.4125, -16.0287) -> (10.3717, -15.9954)
  line L1702 (10.3717, -15.9954) -> (10.3342, -15.9707)
  line L1703 (10.3342, -15.9707) -> (10.3004, -15.9544)
  line L1704 (10.3004, -15.9544) -> (10.2706, -15.9466)
  line L1705 (10.2706, -15.9466) -> (10.2452, -15.9469)
  line L1706 (10.2452, -15.9469) -> (10.2244, -15.9551)
  line L1707 (10.2244, -15.9551) -> (10.196, -15.9733)
  line L1708 (10.196, -15.9733) -> (9.9014, -16.1575)
  line L1709 (9.9014, -16.1575) -> (9.6034, -16.3365)
  line L1710 (9.6034, -16.3365) -> (9.5743, -16.3535)
  line L1711 (9.5743, -16.3535) -> (9.5575, -16.3682)
  line L1712 (9.5575, -16.3682) -> (9.5457, -16.3908)
  line L1713 (9.5457, -16.3908) -> (9.5392, -16.4209)
  line L1714 (9.5392, -16.4209) -> (9.5383, -16.4584)
  line L1715 (9.5383, -16.4584) -> (9.5433, -16.503)
  line L1716 (9.5433, -16.503) -> (9.5545, -16.5545)
  line L1717 (9.5545, -16.5545) -> (9.6038, -16.7112)
  line L1718 (9.6038, -16.7112) -> (9.6574, -16.9003)
  line L1719 (9.6574, -16.9003) -> (9.7107, -17.1235)
  line L1720 (9.7107, -17.1235) -> (9.7608, -17.3806)
  line L1721 (9.7608, -17.3806) -> (9.805, -17.6718)
  line L1722 (9.805, -17.6718) -> (9.8239, -17.8299)
  line L1723 (9.8239, -17.8299) -> (9.8405, -17.9977)
  line L1724 (9.8405, -17.9977) -> (9.8541, -18.1718)
  line L1725 (9.8541, -18.1718) -> (9.8647, -18.3579)
  line L1726 (9.8647, -18.3579) -> (9.8711, -18.5354)
  arc A49 (9.1934, -18.8807) -> (9.8711, -18.5354) centre (0, 0) ccw
  line L1727 (9.1934, -18.8807) -> (9.0535, -18.7712)
  line L1728 (9.0535, -18.7712) -> (8.9092, -18.6532)
  line L1729 (8.9092, -18.6532) -> (8.7763, -18.5399)
  line L1730 (8.7763, -18.5399) -> (8.6503, -18.4279)
  line L1731 (8.6503, -18.4279) -> (8.5336, -18.3196)
  line L1732 (8.5336, -18.3196) -> (8.324, -18.1127)
  line L1733 (8.324, -18.1127) -> (8.1454, -17.9211)
  line L1734 (8.1454, -17.9211) -> (7.9961, -17.7468)
  line L1735 (7.9961, -17.7468) -> (7.8747, -17.5923)
  line L1736 (7.8747, -17.5923) -> (7.7769, -17.4603)
  line L1737 (7.7769, -17.4603) -> (7.7418, -17.4209)
  line L1738 (7.7418, -17.4209) -> (7.7086, -17.3907)
  line L1739 (7.7086, -17.3907) -> (7.6778, -17.3694)
  line L1740 (7.6778, -17.3694) -> (7.6496, -17.3569)
  line L1741 (7.6496, -17.3569) -> (7.6244, -17.3532)
  line L1742 (7.6244, -17.3532) -> (7.6026, -17.3581)
  line L1743 (7.6026, -17.3581) -> (7.5717, -17.3717)
  line L1744 (7.5717, -17.3717) -> (7.2519, -17.5075)
  line L1745 (7.2519, -17.5075) -> (6.9296, -17.6376)
  line L1746 (6.9296, -17.6376) -> (6.8982, -17.6499)
  line L1747 (6.8982, -17.6499) -> (6.8793, -17.6618)
  line L1748 (6.8793, -17.6618) -> (6.8641, -17.6823)
  line L1749 (6.8641, -17.6823) -> (6.853, -17.711)
  line L1750 (6.853, -17.711) -> (6.8462, -17.7479)
  line L1751 (6.8462, -17.7479) -> (6.8442, -17.7927)
  line L1752 (6.8442, -17.7927) -> (6.8472, -17.8454)
  line L1753 (6.8472, -17.8454) -> (6.8714, -18.0079)
  line L1754 (6.8714, -18.0079) -> (6.8947, -18.203)
  line L1755 (6.8947, -18.203) -> (6.9124, -18.4318)
  line L1756 (6.9124, -18.4318) -> (6.9217, -18.6935)
  line L1757 (6.9217, -18.6935) -> (6.9198, -18.9881)
  line L1758 (6.9198, -18.9881) -> (6.9138, -19.1472)
  line L1759 (6.9138, -19.1472) -> (6.9039, -19.3155)
  line L1760 (6.9039, -19.3155) -> (6.8901, -19.4896)
  line L1761 (6.8901, -19.4896) -> (6.8714, -19.675)
  line L1762 (6.8714, -19.675) -> (6.85, -19.8514)
  arc A50 (6.1266, -20.0864) -> (6.85, -19.8514) centre (0, 0) ccw
  line L1763 (6.1266, -20.0864) -> (6.0056, -19.9563)
  line L1764 (6.0056, -19.9563) -> (5.8815, -19.8173)
  line L1765 (5.8815, -19.8173) -> (5.768, -19.6846)
  line L1766 (5.768, -19.6846) -> (5.661, -19.5542)
  line L1767 (5.661, -19.5542) -> (5.5627, -19.429)
  line L1768 (5.5627, -19.429) -> (5.388, -19.1919)
  line L1769 (5.388, -19.1919) -> (5.2416, -18.9746)
  line L1770 (5.2416, -18.9746) -> (5.1215, -18.7791)
  line L1771 (5.1215, -18.7791) -> (5.0257, -18.6076)
  line L1772 (5.0257, -18.6076) -> (4.9497, -18.4619)
  line L1773 (4.9497, -18.4619) -> (4.9212, -18.4175)
  line L1774 (4.9212, -18.4175) -> (4.8932, -18.3825)
  line L1775 (4.8932, -18.3825) -> (4.8661, -18.3566)
  line L1776 (4.8661, -18.3566) -> (4.8402, -18.3399)
  line L1777 (4.8402, -18.3399) -> (4.8159, -18.3323)
  line L1778 (4.8159, -18.3323) -> (4.7936, -18.3337)
  line L1779 (4.7936, -18.3337) -> (4.761, -18.3423)
  line L1780 (4.761, -18.3423) -> (4.4238, -18.4264)
  line L1781 (4.4238, -18.4264) -> (4.0852, -18.5045)
  line L1782 (4.0852, -18.5045) -> (4.0522, -18.5117)
  line L1783 (4.0522, -18.5117) -> (4.0317, -18.5206)
  line L1784 (4.0317, -18.5206) -> (4.0135, -18.5383)
  line L1785 (4.0135, -18.5383) -> (3.998, -18.565)
  line L1786 (3.998, -18.565) -> (3.9856, -18.6004)
  line L1787 (3.9856, -18.6004) -> (3.9765, -18.6443)
  line L1788 (3.9765, -18.6443) -> (3.9713, -18.6968)
  line L1789 (3.9713, -18.6968) -> (3.9697, -18.8611)